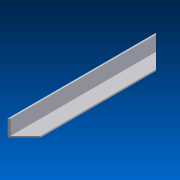
# Autodesk Inventor part: BOXC_L17P5
Saved by Autodesk Inventor 2012 (Build 160160000, 160)
## iProperties
Created: 2012-06-30
Part Number: BOXC_L17P5
Material: Default
Document SubType Name: Modeling
Designer: Hemant
Density: 1 g/cm^3
Author: Hemant
Autodesk Inventor part; units mm, degrees
ref_plane "YZ Plane" through (0, 0, 0) normal (1, 0, 0) x (0, 1, 0)
ref_plane "XZ Plane" through (0, 0, 0) normal (0, 1, 0) x (-1, 0, 0)
ref_plane "XY Plane" through (0, 0, 0) normal (0, 0, 1) x (1, 0, 0)
sketch "Sketch1" plane through (0, 0, 0) normal (0, 0, 1) x (1, 0, 0)
  line L0 (0, 0) -> (0, 50.8)
  line L1 (0, 50.8) -> (4.7625, 50.8)
  line L2 (4.7625, 50.8) -> (4.7625, 4.7625)
  line L3 (4.7625, 4.7625) -> (50.8, 4.7625)
  line L4 (50.8, 4.7625) -> (50.8, 0)
  line L5 (50.8, 0) -> (0, 0)
  dimension "d0" = 4.7625
  dimension "d1" = 50.8
  dimension "d2" = 4.7625
  dimension "d3" = 50.8
  constraints: 12 end point, 4 parallel, 1 perpendicular, 1 vertical
  measures "d0" distance between parallel lines of L2 L0
  measures "d1" distance between parallel lines of L5 L1
  measures "d2" distance between parallel lines of L5 L3
  measures "d3" distance between parallel lines of L4 L0
extrude "Extrusion1" add sketch "Sketch1" along normal blind 457.2
sketch "Sketch5" plane through (0, 0, 0) normal (0, -1, 0) x (1, 0, 0)
  line L0 (50.8, 457.2) -> (0, 457.2) projected
  line L1 (50.8, 0) -> (0, 0) projected
  line L2 (50.8, 0) -> (50.8, 457.2) projected
  line L3 (0, 457.2) -> (50.8, 406.4)
  line L4 (0, 0) -> (50.8, 50.8)
  dimension "d16" = 45
  dimension "d17" = 45
  constraints: 4 end point, 2 point on line
  measures "d16" angle of L3 L0
  measures "d17" angle of L1 L4
extrude "Extrusion5" cut sketch "Sketch5" against normal blind 50.8 contours L2 L3 L0
sketch "Sketch6" plane through (0, 0, 0) normal (0, -1, 0) x (1, 0, 0)
  line L0 (0, 0) -> (0, 457.2) projected
  line L1 (50.8, 0) -> (0, 0) projected
  line L2 (50.8, 0) -> (50.8, 406.4) projected
  line L3 (0, 0) -> (50.8, 50.8)
  dimension "d20" = 45
  constraints: 2 end point, 1 point on line
  measures "d20" angle of L3 L0
extrude "Extrusion6" cut sketch "Sketch6" against normal blind 50.8
body "Solid1"
